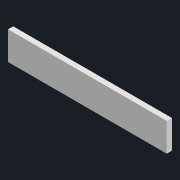
# Autodesk Inventor part: LaminaSoporteAccionador
Saved by Autodesk Inventor 2021 (Build 250183000, 183)
## iProperties
Created: 2021-06-15
Part Number: LaminaSoporteAccionador
Material: Generic
Document SubType Name: Modeling
Designer: GABRIEL LOL
Density: 1 g/cm^3
Appearance: Default
Author: GABRIEL LOL
Autodesk Inventor part; units mm, degrees
ref_plane "YZ Plane" through (0, 0, 0) normal (1, 0, 0) x (0, 1, 0)
ref_plane "XZ Plane" through (0, 0, 0) normal (0, 1, 0) x (-1, 0, 0)
ref_plane "XY Plane" through (0, 0, 0) normal (0, 0, 1) x (1, 0, 0)
sketch "Sketch1" plane through (0, 0, 0) normal (0, 0, 1) x (1, 0, 0)
  line L0 (35.5364, -23.4911) -> (-104.4636, -23.4911)
  line L1 (-104.4636, -23.4911) -> (-104.4636, -48.4911)
  line L2 (-104.4636, -48.4911) -> (35.5364, -48.4911)
  line L3 (35.5364, -48.4911) -> (35.5364, -23.4911)
  point P0 (0, 0)
  dimension "d0" = 140
  dimension "d1" = 25
  constraints: 8 end point, 2 parallel, 1 horizontal, 1 perpendicular
  measures "d0" distance of L2.end L1.end
  measures "d1" distance of L1.end L0.end
extrude "Extrusion1" add sketch "Sketch1" along normal blind 3
sketch "Sketch2" plane through (0, 0, 3) normal (0, 0, 1) x (1, 0, 0)
  line L0 (-37.1754, -34.2701) -> (-113.1754, -34.2701)
  point P0 (0, 0)
  dimension "d5" = 76
  constraints: 2 end point, 1 horizontal
  measures "d5" distance of L0.start L0.end
body "Solid1"
